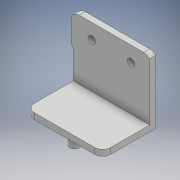
# Autodesk Inventor part: linkageMount
Saved by Autodesk Inventor 2018 (Build 220112000, 112)
## iProperties
Created: 2017-12-31
Part Number: linkageMount
Material: Generic
Document SubType Name: Modeling
Designer: mzhang
Density: 1 g/cm^3
Appearance: Default
Author: mzhang
Autodesk Inventor part; units mm, degrees
ref_plane "YZ Plane" through (0, 0, 0) normal (1, 0, 0) x (0, 1, 0)
ref_plane "XZ Plane" through (0, 0, 0) normal (0, 1, 0) x (-1, 0, 0)
ref_plane "XY Plane" through (0, 0, 0) normal (0, 0, 1) x (1, 0, 0)
sketch "Sketch1" plane through (0, 0, 0) normal (0, 1, 0) x (-1, 0, 0)
  line L0 (0, 0) -> (38.1, 0)
  line L1 (38.1, 0) -> (38.1, -15)
  line L2 (38.1, -15) -> (0, -15)
  line L3 (0, -15) -> (0, 0)
  line L4 (39.1, -16) -> (39.1, 0)
  line L5 (-1, 0) -> (-1, -16)
  line L6 (-1, -16) -> (39.1, -16)
  line L7 (39.1, 0) -> (-1, 0)
  circle A0 centre (28.829, -7.5) radius 1.8415
  circle A1 centre (9.271, -7.5) radius 1.8415
  line L8 (38.1, -15) -> (0, -15)
  line L9 (0, -15) -> (0, -32.85)
  line L10 (0, -32.85) -> (38.1, -32.85)
  line L11 (38.1, -32.85) -> (38.1, -15)
  point P0 (19.05, -15)
  point P1 (38.1, -7.5)
  point P2 (19.05, -7.5)
  dimension "d0" = 15
  dimension "d1" = 38.1
  dimension "d2" = 19.558
  dimension "d5" = 1
  dimension "d6" = 3.683
  dimension "d7" = 3.683
  dimension "d18" = 25.35
  dimension "d19" = 7.5
  constraints: 24 end point, 5 parallel, 3 perpendicular, 2 centre point, 2 coincident, 2 horizontal, 2 midpoint
  measures "d0" distance of L0.end L1.end
  measures "d1" distance of L1.end L2.end
  measures "d2" distance of point (9.271, -7.5) point (28.829, -7.5)
  measures "d5" distance between parallel lines of L1 L4
  measures "d6" diameter of A0
  measures "d7" diameter of A1
  measures "d18" distance from line of point (9.271, -7.5) L10
  measures "d19" distance from line of L0 point (9.271, -7.5)
extrude "Extrusion1" add sketch "Sketch1" along normal blind 3
sketch "Sketch2" plane through (0, 0, -32.85) normal (0, 0, -1) x (-1, 0, 0)
  line L0 (0, 0) -> (0, 3) projected
  line L1 (0, 0) -> (38.1, 0)
  line L2 (38.1, 0) -> (38.1, -18.455)
  line L3 (38.1, -18.455) -> (0, -18.455)
  line L4 (0, -18.455) -> (0, 0)
  circle A0 centre (19.05, -18.455) radius 2.4
  line L5 (38.1, -18.455) -> (0, -18.455)
  line L6 (0, -18.455) -> (0, -23.455)
  line L7 (0, -23.455) -> (38.1, -23.455)
  line L8 (38.1, -23.455) -> (38.1, -18.455)
  dimension "d11" = 18.455
  dimension "d14" = 4.8
  dimension "d15" = 5
  constraints: 16 end point, 4 parallel, 2 horizontal, 2 perpendicular, 1 centre point, 1 midpoint, 1 point on line
  measures "d11" distance of L1.end L2.end
  measures "d14" diameter of A0
  measures "d15" distance of L6.end L5.end
extrude "Extrusion2" add sketch "Sketch2" against normal blind 3
extrude "Extrusion3" add sketch "Sketch2" along normal blind 6 contours A0 L3 | L3 A0
fillet "Fillet1" radius 4 2 edges at (-38.1, -23.455, -31.35) (0, -23.455, -31.35)
fillet "Fillet2" radius 4 2 edges at (-39.1, 1.5, -16) (1, 1.5, -16)
fillet "Fillet3" radius 4 2 edges at (-39.1, 1.5, 0) (1, 1.5, 0)
sketch "Sketch3" plane through (0, 3, 0) normal (0, 1, 0) x (1, 0, 0)
  line L0 (0, 16) -> (0, 29.85) projected
  line L1 (13.4327, 0) -> (0, 0)
  line L2 (0, 0) -> (0, 21.087)
  line L3 (0, 21.087) -> (13.4327, 21.087)
  line L4 (13.4327, 21.087) -> (13.4327, 0)
  point P0 (0, 0)
  constraints: 8 end point, 2 parallel, 1 horizontal, 1 perpendicular, 1 point on line
extrude "Extrusion4" cut sketch "Sketch3" against normal up to surface (3 mm away)
body "Solid1"
